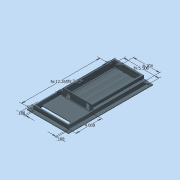
# Autodesk Inventor part: BatteryBox
Saved by Autodesk Inventor 2015 (Build 190159000, 159)
## iProperties
Created: 2015-10-11
Part Number: BatteryBox
Material: ABS Plastic
Document SubType Name: Modeling
Designer: Raphael
Density: 1.06 g/cm^3
Appearance: Lead
Author: Raphael
Autodesk Inventor part; units mm, degrees
ref_plane "YZ Plane" through (0, 0, 0) normal (1, 0, 0) x (0, 1, 0)
ref_plane "XZ Plane" through (0, 0, 0) normal (0, 1, 0) x (-1, 0, 0)
ref_plane "XY Plane" through (0, 0, 0) normal (0, 0, 1) x (1, 0, 0)
sketch "Sketch1" plane through (0, 0, 0) normal (0, 1, 0) x (-1, 0, 0)
  line L0 (0, 0) -> (139.7, 0)
  line L1 (139.7, 0) -> (139.7, -311.5225)
  line L2 (139.7, -311.5225) -> (0, -311.5225)
  line L3 (0, -311.5225) -> (0, 0)
  line L4 (4.7625, -4.7625) -> (134.9375, -4.7625)
  line L5 (134.9375, -4.7625) -> (134.9375, -106.3625)
  line L6 (134.9375, -106.3625) -> (4.7625, -106.3625)
  line L7 (4.7625, -106.3625) -> (4.7625, -4.7625)
  line L8 (121.977, -109.5375) -> (17.723, -109.5375)
  line L9 (17.723, -109.5375) -> (17.723, -305.1725)
  line L10 (17.723, -305.1725) -> (121.977, -305.1725)
  line L11 (121.977, -305.1725) -> (121.977, -109.5375)
  line L12 (128.327, -106.3625) -> (128.327, -311.5225)
  line L13 (11.373, -106.3625) -> (11.373, -311.5225)
  point P0 (69.85, -305.1725)
  point P1 (69.85, -311.5225)
  dimension "d0" = 139.7
  dimension "d1" = 311.5225
  dimension "d2" = 4.7625
  dimension "d3" = 4.7625
  dimension "d4" = 4.7625
  dimension "d5" = 101.6
  dimension "d6" = 104.254
  dimension "d7" = 6.35
  dimension "d8" = 195.635
  dimension "d9" = 6.35
  dimension "d10" = 6.35
  constraints: 28 end point, 6 parallel, 5 perpendicular, 4 point on line, 3 horizontal, 2 midpoint, 1 vertical alignment
  measures "d0" distance of L1.end L2.end
  measures "d1" distance of L0.end L1.end
  measures "d2" distance between parallel lines of L3 L7
  measures "d3" distance between parallel lines of L1 L5
  measures "d4" distance between parallel lines of L0 L4
  measures "d5" distance of L4.end L5.end
  measures "d6" distance of L8.start L8.end
  measures "d7" distance between parallel lines of L2 L10
  measures "d8" distance of L10.end L8.start
  measures "d9" distance between parallel lines of L12 L11
  measures "d10" distance between parallel lines of L9 L13
extrude "Extrusion1" add sketch "Sketch1" along normal blind 29.175 contours L13 L6 L12 L2
extrude "Extrusion2" add sketch "Sketch1" along normal blind 4.7625 contours L11 L10 L9 L8
extrude "Extrusion3" add sketch "Sketch1" along normal blind 3.175 contours L6 L7 L4 L5
extrude "Extrusion4" add sketch "Sketch1" along normal blind 17.4625 contours L0 L1 L2 L12 L6 L5 L4 L7 L13 L3
sketch "Sketch2" plane through (-121.977, 29.175, -305.1725) normal (0, 0, 1) x (1, 0, 0)
  circle A0 centre (13.127, -13) radius 13
  circle A1 centre (39.127, -13) radius 13
  circle A2 centre (65.127, -13) radius 13
  circle A3 centre (91.127, -13) radius 13
  line L0 (-6.35, 0) -> (110.604, 0) projected
  point P0 (121.977, -29.175)
  point P1 (52.127, -13)
  point P2 (52.127, 0)
  dimension "d20" = 26
  dimension "d21" = 26
  dimension "d19" = 26
  dimension "d22" = 26
  constraints: 5 horizontal alignment, 2 centre point, 1 midpoint, 1 tangent, 1 vertical alignment, 6 other
  measures "d19" diameter of A0
  measures "d22" diameter of A3
extrude "Extrusion5" cut sketch "Sketch2" along normal up to surface (195.635 mm away) contours A0 | A1 | A2 | A3
sketch "Sketch3" plane through (-17.723, 29.175, -109.5375) normal (0, 0, -1) x (-1, 0, 0)
  arc A0 (84.9017, -24.4125) -> (97.3523, -24.4125) centre (91.127, -13) ccw projected
  arc A1 (6.9017, -24.4125) -> (19.3523, -24.4125) centre (13.127, -13) ccw projected
  arc A2 (99.0645, -13) -> (83.1895, -13) centre (91.127, -13) ccw
  arc A3 (21.0645, -13) -> (5.1895, -13) centre (13.127, -13) ccw
  line L0 (97.3523, -24.4125) -> (104.254, -24.4125) projected
  line L1 (71.3523, -24.4125) -> (84.9017, -24.4125) projected
  line L2 (0, -24.4125) -> (6.9017, -24.4125) projected
  line L3 (19.3523, -24.4125) -> (32.9017, -24.4125) projected
  line L4 (99.0645, -13) -> (99.0645, -24.4125)
  line L5 (83.1895, -13) -> (83.1895, -24.4125)
  line L6 (21.0645, -13) -> (21.0645, -24.4125)
  line L7 (5.1895, -13) -> (5.1895, -24.4125)
  line L8 (99.0645, -24.4125) -> (83.1895, -24.4125)
  line L9 (-12.9605, -26) -> (117.2145, -26) projected
  line L10 (5.1895, -24.4125) -> (21.0645, -24.4125)
  point P0 (-17.723, -29.175)
  dimension "d25" = 15.875
  dimension "d26" = 15.875
  constraints: 12 end point, 4 point on circle, 4 point on line, 2 centre point, 2 coincident, 2 parallel, 2 perpendicular, 1 collinear, 1 vertical
  measures "d25" diameter of A2
  measures "d26" diameter of A3
extrude "Extrusion6" cut sketch "Sketch3" against normal up to surface (3.175 mm away) contours L1 L5 A2 L4 L0 L8 | L2 L7 A3 L6 L3 L10
sketch "Sketch5" plane through (0, 0, 0) normal (0, -1, 0) x (1, 0, 0)
  line L0 (12.7, 12.7) -> (-152.4, 12.7)
  line L1 (-152.4, 12.7) -> (-152.4, -324.2225)
  line L2 (-152.4, -324.2225) -> (12.7, -324.2225)
  line L3 (12.7, -324.2225) -> (12.7, 12.7)
  line L4 (0, 0) -> (0, -311.5225) projected
  line L5 (-139.7, 0) -> (0, 0) projected
  line L6 (-139.7, -311.5225) -> (-139.7, 0) projected
  line L7 (0, -311.5225) -> (-139.7, -311.5225) projected
  dimension "d32" = 12.7
  dimension "d33" = 12.7
  dimension "d34" = 12.7
  dimension "d35" = 12.7
  constraints: 8 end point, 2 parallel, 1 horizontal, 1 perpendicular
  measures "d32" distance between parallel lines of L7 L2
  measures "d33" distance between parallel lines of L3 L4
  measures "d34" distance between parallel lines of L0 L5
  measures "d35" distance between parallel lines of L6 L1
extrude "Extrusion8" add sketch "Sketch5" against normal blind 3.175 contours L3 L2 L1 L0 | L4 L7 L6 L5
sketch "Sketch4" plane through (0, 3.175, 0) normal (0, 1, 0) x (1, 0, 0)
  line L0 (-4.7625, 4.7625) -> (-4.7625, 106.3625) projected
  line L1 (-4.7625, 106.3625) -> (-134.9375, 106.3625) projected
  line L2 (-134.9375, 106.3625) -> (-134.9375, 4.7625) projected
  line L3 (-134.9375, 4.7625) -> (-4.7625, 4.7625) projected
  line L4 (-134.9375, 4.7625) -> (-134.9375, 106.3625) projected
  line L5 (-134.9375, 30.1625) -> (-4.7625, 30.1625)
  line L6 (-4.7625, 4.7625) -> (-4.7625, 106.3625) projected
  line L7 (-134.9375, 30.1625) -> (-134.9375, 4.7625)
  line L8 (-4.7625, 4.7625) -> (-4.7625, 30.1625)
  line L9 (-4.7625, 4.7625) -> (-134.9375, 4.7625)
  line L10 (-134.9375, 4.7625) -> (-4.7625, 4.7625) projected
  point P0 (0, 0)
  dimension "d29" = 25.4
  constraints: 8 end point, 3 collinear, 2 point on line, 1 perpendicular
  measures "d29" distance between parallel lines of L5 L3
extrude "Extrusion7" cut sketch "Sketch4" against normal blind 17.4625 contours L3 L2 L5 L0
equation "\"d0\" = width"
equation "\"d1\" = length"
equation "\"d8\" = battery_length"
equation "\"d11\" = height"
equation "\"d13\" = bottom_thickness"
equation "\"width\" = 139.7"
equation "\"bottom_thickness\" = 4.7625"
equation "\"battery_length\" = 195.635"
equation "\"length\" = 311.5225"
equation "\"height\" = 29.175"
body "Solid1"
